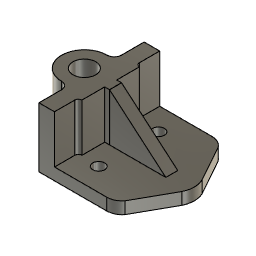
A3 (Autodesk Fusion 360 design; units mm, degrees)
Autodesk Fusion 360 part; units mm, degrees
sketch "Sketch1" plane through (0, 0, 0) normal (0, 0, 1) x (1, 0, 0)
  line L0 (-33.5, 44) -> (33.5, 44)
  line L1 (33.5, -44) -> (-33.5, -44)
  arc A0 (33.5, -19) -> (33.5, 19) centre (33.5, 0) ccw
  line L2 (33.5, 44) -> (33.5, 19)
  line L3 (33.5, -19) -> (33.5, -44)
  line L4 (33.5, 44) -> (-2.5, 44) construction
  line L5 (2.5, -25) -> (33.5, -25) construction
  line L6 (33.5, -25) -> (-20, -25) construction
  circle A1 centre (-2.5, 25) radius 5 construction
  circle A2 centre (-2.5, -25) radius 5 construction
  circle A3 centre (-2.5, -25) radius 5
  circle A4 centre (-2.5, 25) radius 5
  line L7 (-33.5, 44) -> (-20.5, 44)
  line L8 (-20.5, 44) -> (-39.5, 44)
  line L9 (0, 0) -> (-90, 0) construction
  circle A5 centre (-39.5, 0) radius 9.5 construction
  circle A6 centre (-39.5, 0) radius 9.5
  line L10 (-33.5, -44) -> (-33.5, -18.0278)
  line L11 (-33.5, 18.0278) -> (-33.5, 44)
  arc A7 (-33.5, 18.0278) -> (-33.5, -18.0278) centre (-39.5, 0) ccw
  dimension "d10" = 19
  dimension "d12" = 10
  dimension "d13" = 10
  dimension "d14" = 13
  dimension "d15" = 19
  dimension "d16" = 19
  dimension "d17" = 19
  constraint horizontal L0
  constraint perpendicular L0 L2
  constraint parallel L0 L1
  constraint parallel L2 L10
  constraint coincident L9.start origin
  constraint coincident A0.start L2
  constraint collinear L2 L3
  constraint coincident A0.centre L2
  constraint perpendicular L2 L4
  constraint coincident L3 L5.end
  constraint perpendicular L3 L5
  constraint perpendicular L3 L6
  constraint coincident L6 A2.centre
  constraint concentric A2 A3
  constraint concentric A1 A4
  constraint perpendicular L7 L10
  constraint parallel L0 L8
  constraint horizontal L9
  constraint coincident L9 A5.centre
  constraint concentric A5 A6
  constraint concentric A6 A7
  constraint collinear L10 L11
  measures "d10" radius of A0
  measures "d12" diameter of A1
  measures "d13" diameter of A2
  measures "d14" distance of L0.start L7.end
  measures "d15" distance of L7.end L8.end
  measures "d16" diameter of A5
  measures "d17" radius of A7
extrude "Extrude1" add sketch "Sketch1" along normal blind 10
chamfer "Chamfer1" distance 20 angle 45 2 edges at (33.5, -19, 5) (33.5, 19, 5)
fillet "Fillet1" radius 13 2 edges at (33.5, -44, 5) (33.5, 44, 5)
sketch "Sketch2" plane through (0, 0, 10) normal (0, 0, 1) x (-1, 0, 0)
  arc A0 (-33.5, -39) -> (-23.253, -44) centre (-23.253, -31) ccw
  line L0 (-23.253, -44) -> (33.5, -44)
  line L1 (33.5, -44) -> (33.5, -18.0278)
  arc A1 (33.5, -18.0278) -> (33.5, 18.0278) centre (39.5, 0) ccw
  line L2 (33.5, 18.0278) -> (33.5, 44)
  line L3 (33.5, 44) -> (-23.253, 44)
  arc A2 (-23.253, 44) -> (-33.5, 39) centre (-23.253, 31) ccw
  line L4 (-33.5, 39) -> (-50.5058, 8.4737)
  arc A3 (-50.5058, 8.4737) -> (-50.5058, -8.4737) centre (-33.5, 0) ccw
  line L5 (-50.5058, -8.4737) -> (-33.5, -39)
  circle A4 centre (39.5, 0) radius 9.5
  circle A5 centre (2.5, -25) radius 5
  circle A6 centre (2.5, 25) radius 5
  line L6 (33.5, -44) -> (20.5, -44)
  line L7 (33.5, -44) -> (33.5, -18.0278)
  line L8 (33.5, 18.0278) -> (33.5, 44)
  line L9 (33.5, 44) -> (20.5, 44)
  circle A7 centre (39.5, 0) radius 9.5
  arc A8 (33.5, -18.0278) -> (33.5, 18.0278) centre (39.5, 0) ccw
  line L10 (33.5, -44) -> (13.5, -44) construction
  line L11 (13.5, 0) -> (13.5, -5)
  line L12 (13.5, 0) -> (13.5, 5)
  line L13 (13.5, -5) -> (17.5, -5)
  line L14 (13.5, 5) -> (17.5, 5)
  line L15 (17.5, -5) -> (17.5, -24)
  line L16 (17.5, 5) -> (17.5, 24)
  line L17 (20.5, 44) -> (20.5, 24)
  line L18 (20.5, -44) -> (20.5, -24)
  line L19 (17.5, -24) -> (20.5, -24)
  line L20 (20.5, 24) -> (17.5, 24)
  dimension "d23" = 13
  dimension "d24" = 13
  dimension "d25" = 20
  constraint coincident L0.end L1.start
  constraint perpendicular L1 L6
  constraint coincident L1.end A1.start
  constraint coincident A1.end L2.start
  constraint coincident L2.end L3.start
  constraint perpendicular L2 L9
  constraint concentric A1 A7
  constraint concentric A7 A8
  constraint perpendicular L7 L10
  constraint perpendicular L11 L13
  constraint perpendicular L12 L14
  constraint perpendicular L13 L15
  constraint perpendicular L14 L16
  constraint perpendicular L9 L17
  constraint perpendicular L10 L18
  constraint perpendicular L18 L19
  constraint perpendicular L16 L20
  measures "d23" distance of L0.end L6.end
  measures "d24" distance of L2.end L9.end
  measures "d25" distance of L0.end L10.end
extrude "Extrude2" add sketch "Sketch2" along normal blind 40 contours L0 L1 A1 L2 L3 L6 L7 L8 L9 A8 L11 L12 L13 L14 L15 L16 L17 L18 L19 L20
fillet "Fillet2" radius 3 1 edges at (-20.5, -24, 30)
fillet "Fillet3" radius 3 1 edges at (-20.5, 24, 30)
fillet "Fillet4" radius 6 2 edges at (-33.5, -18.0278, 25) (-33.5, 18.0278, 25)
sketch "Sketch3" plane through (0, 0, 0) normal (0, 1, 0) x (1, 0, 0)
  line L0 (-13.4027, -9.9935) -> (33.5973, -9.9935)
  line L1 (-13.4027, -9.9935) -> (-13.4027, -49.9935)
  line L2 (-13.4027, -49.9935) -> (33.5973, -9.9935)
  dimension "d40" = 47
  constraint horizontal L0
  constraint perpendicular L0 L1
  measures "d40" distance of L0.start L0.end
extrude "Extrude3" add sketch "Sketch3" along normal mid plane 10
